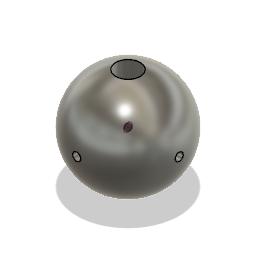
_sphere.aaea48cb-db7c-48fc-b7af-8c36bddd8de9 (Autodesk Fusion 360 design; units mm, degrees)
Autodesk Fusion 360 part; units mm, degrees
sphere "SpherePrimitive1" add diameter 38 placed x (1, 0, 0) y (0, 0, -1) z (0, 1, 0) at (0, 0, 0)
sketch "Sketch2" plane through (0, 0, 0) normal (1, 0, 0) x (0, 0, -1)
  circle A0 centre (0, 0) radius 1.5
  dimension "d2" = 3
  measures "d2" diameter of A0
sketch "Sketch3" plane through (0, 0, 0) normal (0, 0, 1) x (1, 0, 0)
  circle A0 centre (0, 0) radius 1.5
  dimension "d3" = 3
  measures "d3" diameter of A0
sketch "Sketch4" plane through (0, 0, 0) normal (0, 1, 0) x (1, 0, 0)
  circle A0 centre (0, 0) radius 4.5
  dimension "d4" = 9
  measures "d4" diameter of A0
extrude "Extrude1" cut sketch "Sketch4" along normal blind 50
extrude "Extrude2" cut sketch "Sketch2" along normal mid plane 100
extrude "Extrude3" cut sketch "Sketch3" along normal mid plane 120
